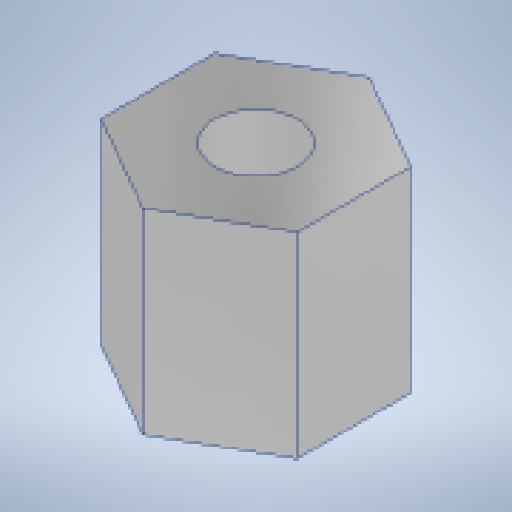
# Autodesk Inventor part: basespacer1
Saved by Autodesk Inventor 2024.3 (Build 283343010, 343A)
## iProperties
Created: 2025-10-01
Part Number: basespacer1
Material: アルミニウム 6061
Document SubType Name: Modeling
Designer: kshau
Density: 2.7 g/cm^3
Appearance: アルミニウム - フラット
Author: kshau
Autodesk Inventor part; units mm, degrees
ref_plane "YZ Plane" through (0, 0, 0) normal (1, 0, 0) x (0, 1, 0)
ref_plane "XZ Plane" through (0, 0, 0) normal (0, 1, 0) x (-1, 0, 0)
ref_plane "XY Plane" through (0, 0, 0) normal (0, 0, 1) x (1, 0, 0)
sketch "スケッチ1" plane through (0, 0, 0) normal (0, 1, 0) x (-1, 0, 0)
  circle A0 centre (0, 0) radius 5.7735
  line L0 (0, 0) -> (5, -2.8868)
  line L1 (5, -2.8868) -> (5, 0)
  line L2 (0, 0) -> (5, 0)
  line L3 (5, 2.8868) -> (5, 0)
  line L4 (5, 2.8868) -> (2.5, 4.3301)
  line L5 (0, 5.7735) -> (2.5, 4.3301)
  line L6 (0, 5.7735) -> (-2.5, 4.3301)
  line L7 (-5, 2.8868) -> (-2.5, 4.3301)
  line L8 (-5, 2.8868) -> (-5, 0)
  line L9 (-5, -2.8868) -> (-5, 0)
  line L10 (-5, -2.8868) -> (-2.5, -4.3301)
  line L11 (0, -5.7735) -> (-2.5, -4.3301)
  line L12 (0, -5.7735) -> (2.5, -4.3301)
  line L13 (5, -2.8868) -> (2.5, -4.3301)
  dimension "d1" = 5
  dimension "d2" = 30
  dimension "d5" = 360
  constraints: 28 end point, 1 coincident, 1 horizontal, 1 symmetric about line, 1 vertical, 34 other
  measures "d1" distance from line of point (0, 0) L1
  measures "d2" angle of L2 L0
extrude "押し出し1" add sketch "スケッチ1" along normal blind 10 contours L3 L2 L0 L13 L12 L11 L10 L9 L8 L7 L6 L5 L4 | L0 L2 L1
sketch "スケッチ2" plane through (0, 10, 0) normal (0, 1, 0) x (1, 0, 0)
  point P0 (0, 0)
  point P1 (0, 0)
  constraints: 1 coincident
hole "穴1" at (0, 10, 0) direction (0, -1, 0) diameter 4.2 end through all
